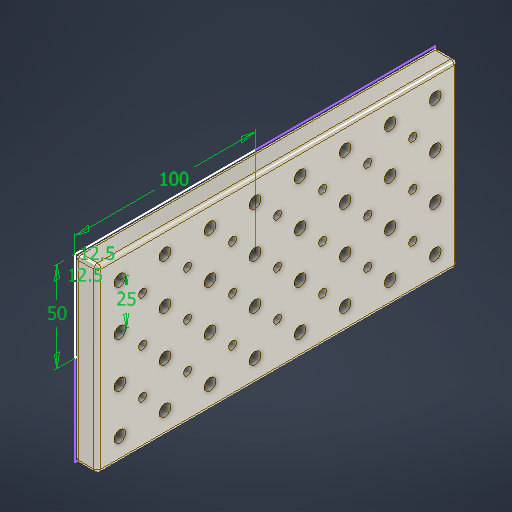
# Autodesk Inventor part: Mount
Saved by Autodesk Inventor 2027 (Build 310192060, 192F)
## iProperties
Created: 2026-05-22
Part Number: Mount
Material: Titanium
Document SubType Name: Modeling
Designer: jacob
Density: 4.51 g/cm^3
Appearance: Titanium
Author: jacob
Autodesk Inventor part; units mm, degrees
ref_plane "YZ Plane" through (0, 0, 0) normal (1, 0, 0) x (0, 1, 0)
ref_plane "XZ Plane" through (0, 0, 0) normal (0, 1, 0) x (-1, 0, 0)
ref_plane "XY Plane" through (0, 0, 0) normal (0, 0, 1) x (1, 0, 0)
sketch "fourth" plane through (0, 0, 0) normal (1, 0, 0) x (0, 1, 0)
  line L0 (50, 100) -> (50, 0)
  line L1 (50, 100) -> (0, 100)
  line L2 (0, 75) -> (0, 100)
  line L3 (0, 75) -> (0, 50)
  line L4 (0, 50) -> (0, 25)
  line L5 (0, 25) -> (0, 0)
  line L6 (25, 75) -> (0, 75)
  line L7 (25, 75) -> (25, 50)
  line L8 (25, 50) -> (25, 25)
  line L9 (25, 25) -> (25, 0)
  line L10 (37.5, 87.5) -> (37.5, 62.5)
  line L11 (37.5, 62.5) -> (37.5, 37.5)
  line L12 (37.5, 37.5) -> (37.5, 12.5)
  line L13 (12.5, 87.5) -> (37.5, 87.5)
  line L14 (12.5, 87.5) -> (12.5, 62.5)
  line L15 (12.5, 62.5) -> (12.5, 37.5)
  line L16 (12.5, 37.5) -> (12.5, 12.5)
  line L17 (50, -100) -> (50, 0)
  line L18 (50, -100) -> (0, -100)
  line L19 (0, -75) -> (0, -100)
  line L20 (0, -75) -> (0, -50)
  line L21 (0, -50) -> (0, -25)
  line L22 (0, -25) -> (0, 0)
  line L23 (25, -75) -> (0, -75)
  line L24 (25, -75) -> (25, -50)
  line L25 (25, -50) -> (25, -25)
  line L26 (25, -25) -> (25, 0)
  line L27 (37.5, -87.5) -> (37.5, -62.5)
  line L28 (37.5, -62.5) -> (37.5, -37.5)
  line L29 (37.5, -37.5) -> (37.5, -12.5)
  line L30 (12.5, -87.5) -> (37.5, -87.5)
  line L31 (12.5, -87.5) -> (12.5, -62.5)
  line L32 (12.5, -62.5) -> (12.5, -37.5)
  line L33 (12.5, -37.5) -> (12.5, -12.5)
  line L34 (-50, 100) -> (-50, 0)
  line L35 (-50, 100) -> (0, 100)
  line L36 (-25, 75) -> (0, 75)
  line L37 (-25, 75) -> (-25, 50)
  line L38 (-25, 50) -> (-25, 25)
  line L39 (-25, 25) -> (-25, 0)
  line L40 (-37.5, 87.5) -> (-37.5, 62.5)
  line L41 (-37.5, 62.5) -> (-37.5, 37.5)
  line L42 (-37.5, 37.5) -> (-37.5, 12.5)
  line L43 (-12.5, 87.5) -> (-37.5, 87.5)
  line L44 (-12.5, 87.5) -> (-12.5, 62.5)
  line L45 (-12.5, 62.5) -> (-12.5, 37.5)
  line L46 (-12.5, 37.5) -> (-12.5, 12.5)
  line L47 (-25, -75) -> (-25, -50)
  line L48 (-25, -75) -> (0, -75)
  line L49 (-37.5, -87.5) -> (-37.5, -62.5)
  line L50 (-12.5, -87.5) -> (-12.5, -62.5)
  line L51 (-50, -100) -> (0, -100)
  line L52 (-12.5, -87.5) -> (-37.5, -87.5)
  line L53 (-37.5, -62.5) -> (-37.5, -37.5)
  line L54 (-12.5, -62.5) -> (-12.5, -37.5)
  line L55 (-50, -100) -> (-50, 0)
  line L56 (-25, -50) -> (-25, -25)
  line L57 (-37.5, -37.5) -> (-37.5, -12.5)
  line L58 (-12.5, -37.5) -> (-12.5, -12.5)
  line L59 (-25, -25) -> (-25, 0)
  dimension "d16" = 50
  dimension "d22" = 100
  dimension "d23" = 100
  dimension "d24" = 25
  dimension "d25" = 12.5
  dimension "d26" = 12.5
  constraints: 120 end point, 7 collinear, 6 equal length, 5 vertical, 2 horizontal, 1 coincident, 1 perpendicular
  measures "d16" distance of L0.start L1.end
  measures "d22" distance of L0.start L0.end
  measures "d23" vertical distance of point (0, 0) L0.start
  measures "d24" distance of L6.start L2.start
  measures "d25" distance from line of L0 L10.start
  measures "d26" distance from line of L1 L10.start
extrude "Extrusion1" add sketch "fourth" along normal blind 12.5
hole "Hole1" at (0, 25, 75) at (0, 25, 50) at (0, 25, 25) at (0, 25, 0) at (0, 25, -25) at (0, 25, -50) at (0, 25, -75) at (0, 0, 75) at (0, 0, 50) at (0, -25, 75) at (0, -25, 50) at (0, -25, 25) at (0, -25, 0) at (0, -25, -25) at (0, -25, -50) at (0, -25, -75) at (0, 0, -75) at (0, 0, -50) at (0, 0, -25) at (0, 0, 0) at (0, 0, 25) direction (1, 0, 0) diameter 4.5 end through all
hole "Hole2" at (0, 37.5, 87.5) at (0, 37.5, 62.5) at (0, 37.5, 37.5) at (0, 37.5, 12.5) at (0, 12.5, 87.5) at (0, 12.5, 62.5) at (0, 12.5, 37.5) at (0, 12.5, 12.5) at (0, 37.5, -87.5) at (0, 37.5, -62.5) at (0, 12.5, -87.5) at (0, 12.5, -62.5) at (0, 37.5, -37.5) at (0, 12.5, -37.5) at (0, 37.5, -12.5) at (0, 12.5, -12.5) at (0, -37.5, 87.5) at (0, -37.5, 62.5) at (0, -37.5, 37.5) at (0, -37.5, 12.5) at (0, -12.5, 37.5) at (0, -12.5, 12.5) at (0, -12.5, 62.5) at (0, -12.5, 87.5) at (0, -37.5, -37.5) at (0, -37.5, -12.5) at (0, -12.5, -37.5) at (0, -12.5, -12.5) at (0, -37.5, -62.5) at (0, -12.5, -62.5) at (0, -12.5, -87.5) at (0, -37.5, -87.5) direction (1, 0, 0) diameter 6.5 end through all
fillet "Fillet1" radius 2 12 edges at (12.5, 0, 100) (12.5, 50, 0) (12.5, 0, -100) (12.5, -50, 0) (0, 50, 0) (0, 0, 100) (0, -50, 0) (0, 0, -100) (6.25, 50, -100) (6.25, 50, 100) (6.25, -50, 100) (6.25, -50, -100)
body "Solid1"
